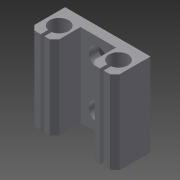
# Autodesk Inventor part: XCarriageV7
Saved by Autodesk Inventor 2015 (Build 190159000, 159)
## iProperties
Created: 2014-08-21
Part Number: XCarriageV7
Material: Generic
Document SubType Name: Modeling
Designer: t_clevj
Density: 1 g/cm^3
Appearance: Default
Author: t_clevj
Autodesk Inventor part; units mm, degrees
ref_plane "YZ Plane" through (0, 0, 0) normal (1, 0, 0) x (0, 1, 0)
ref_plane "XZ Plane" through (0, 0, 0) normal (0, 1, 0) x (-1, 0, 0)
ref_plane "XY Plane" through (0, 0, 0) normal (0, 0, 1) x (1, 0, 0)
sketch "Sketch1" plane through (0, 0, 0) normal (0, 0, 1) x (1, 0, 0)
  circle A0 centre (0, 0) radius 8
  circle A1 centre (50, 0) radius 8
  line L0 (-1.5, -7.8581) -> (-1.5, -14)
  line L1 (-1.5, -14) -> (-11, -14)
  line L2 (-11, -14) -> (-11, 16)
  line L3 (-11, 16) -> (61, 16)
  line L4 (61, 16) -> (61, -14)
  line L5 (61, -14) -> (51.5, -14)
  line L6 (51.5, -14) -> (51.5, -7.8581)
  line L7 (48.5, -7.8581) -> (48.5, -14)
  line L8 (48.5, -14) -> (40, -14)
  line L9 (40, -14) -> (40, 8)
  line L10 (40, 8) -> (10, 8)
  line L11 (10, 8) -> (10, -14)
  line L12 (10, -14) -> (1.5, -14)
  line L13 (1.5, -14) -> (1.5, -7.8581)
  dimension "d0" = 16
  dimension "d1" = 16
  dimension "d2" = 50
  dimension "d3" = 1.5
  dimension "d4" = 1.5
  dimension "d5" = 1.5
  dimension "d6" = 1.5
  dimension "d7" = 14
  dimension "d8" = 10
  dimension "d9" = 10
  dimension "d10" = 8
  dimension "d11" = 11
  dimension "d12" = 11
  dimension "d13" = 8
  constraints: 28 end point, 10 perpendicular, 4 horizontal alignment, 4 point on circle, 4 point on line, 2 centre point, 2 vertical, 1 coincident
  measures "d0" diameter of A0
  measures "d1" diameter of A1
  measures "d2" distance of A1.centre point (0, 0)
  measures "d3" distance from line of point (0, 0) L13
  measures "d4" distance from line of point (0, 0) L0
  measures "d5" distance from line of A1.centre L7
  measures "d6" distance from line of A1.centre L6
  measures "d7" distance from line of point (0, 0) L12
  measures "d8" distance from line of point (0, 0) L11
  measures "d9" distance from line of A1.centre L9
  measures "d10" distance between parallel lines of L3 L10
  measures "d11" distance from line of A1.centre L4
  measures "d12" distance from line of L2 point (0, 0)
  measures "d13" distance from line of A1.centre L10
extrude "Extrusion1" add sketch "Sketch1" along normal blind 70 contours A0 L0 L1 L2 L3 L4 L5 L6 A1 L7 L8 L9 L10 L11 L12 L13
chamfer "Chamfer1" distance 4 angle 45 4 edges at (-11, -14, 35) (10, -14, 35) (40, -14, 35) (61, -14, 35)
sketch "Sketch2" plane through (10, 8, 0) normal (0, -1, 0) x (1, 0, 0)
  line L0 (0, 0) -> (30, 0) projected
  line L1 (30, 0) -> (30, 70) projected
  circle A0 centre (15, 55) radius 8
  circle A1 centre (15, 15) radius 8
  point P0 (-10, 0)
  dimension "d19" = 16
  dimension "d20" = 16
  dimension "d21" = 40
  dimension "d22" = 15
  dimension "d23" = 15
  constraints: 2 centre point, 1 vertical alignment
  measures "d19" diameter of A0
  measures "d20" diameter of A1
  measures "d21" distance of A0.centre A1.centre
  measures "d22" distance from line of L0 A1.centre
  measures "d23" distance from line of L1 A1.centre
extrude "Extrusion2" cut sketch "Sketch2" against normal up to surface (8 mm away)
body "Solid1"
